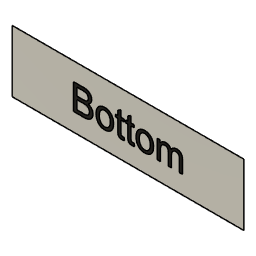
bottom_label (Autodesk Fusion 360 design; units mm, degrees)
part number: 2025-04-13-10-14-33-970
Autodesk Fusion 360 part; units mm, degrees
sketch "Sticker" plane through (0, 0, 0) normal (0, 1, 0) x (1, 0, 0)
  line L0 (0, 0) -> (45, 0)
  line L1 (45, 0) -> (45, -12)
  line L2 (45, -12) -> (0, -12)
  line L3 (0, -12) -> (0, 0)
  dimension "d1" = 12
  dimension "d2" = 45
  constraint horizontal L0
  constraint vertical L1
  constraint horizontal L2
  constraint vertical L3
  constraint coincident L0.start L3.end
  measures "d1" distance of L0.end L1.end
  measures "d2" distance of L0.start L0.end
extrude "Extrude1" add sketch "Sticker" along normal blind 0.01 makes body 1
sketch "Text" plane through (0, 0, 0) normal (0, -1, 0) x (1, 0, 0)
  line L0 (45, 12) -> (0, 12)
  line L1 (0, 12) -> (0, 0)
  line L2 (0, 0) -> (45, 0)
  line L3 (45, 0) -> (45, 12)
  line L4 (0, 0) -> (45, 0) construction
  line L5 (45, 0) -> (45, 12) construction
  line L6 (45, 12) -> (0, 12) construction
  line L7 (0, 12) -> (0, 0) construction
  dimension "d5" = 5
  text T0 "Bottom" font "Arial" height 5 align centre middle in box 45 x 12 at (0, 0) x (1, 0) y (0, 1) spacing 1 kerned
  constraint coincident L2.end
  constraint coincident L0.end
extrude "Extrude2" add sketch "Text" along normal blind 0.01 separate body text T0 makes body 2 at (16.525, 0, 5.5613) makes body 3 at (28.3799, 0, 5.3338) makes body 4 at (24.291, 0, 5.5613) makes body 5 at (22.8695, 0, 5.244) makes body 6 at (20.9288, 0, 5.244) makes body 7 at (12.1373, 0, 5.9363)
named bodies: "Sticker", "Text 2", "Text 6", "Text 5", "Text 4", "Text 3", "Text 1"
